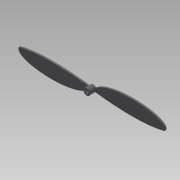
# Autodesk Inventor part: Helice 7x3
Saved by Autodesk Inventor 2016 (Build 200138000, 138)
## iProperties
Created: 2016-01-22
Part Number: Helice 7x3
Material: Plastique ABS
Document SubType Name: Modeling
Designer: sd
Density: 1.06 g/cm^3
Appearance: Lisse - Gris moyen
Mass: 5.43361 g
Surface Area: 59.4069 cm^2
Volume: 5.12605 cm^3
Author: sd
Autodesk Inventor part; units mm, degrees
ref_plane "YZ Plane" through (0, 0, 0) normal (1, 0, 0) x (0, 1, 0)
ref_plane "XZ Plane" through (0, 0, 0) normal (0, 1, 0) x (-1, 0, 0)
ref_plane "XY Plane" through (0, 0, 0) normal (0, 0, 1) x (1, 0, 0)
sketch "Esquisse4" plane through (0, 0, 0) normal (0, 1, 0) x (-1, 0, 0)
  circle A0 centre (0, 0) radius 2.25
  circle A1 centre (0, 0) radius 4
  dimension "d6" = 4.5
  dimension "d7" = 8
  constraints: 2 centre point, 2 coincident
  measures "d6" diameter of A0
  measures "d7" diameter of A1
extrude "Extrusion2" add sketch "Esquisse4" along normal blind 8
sketch "Esquisse5" plane through (0, 8, 0) normal (0, 1, 0) x (1, 0, 0)
  circle A0 centre (0, 0) radius 4 projected
  circle A1 centre (0, 0) radius 88.9
  spline S0 degree 3 poles (-88.9, 0) (-96.1137, 15.1507) (-22.3547, 20.9921) (-3.3072, 2.25) knots 0 0 0 0 1 1 1 1
  spline S1 degree 2 poles (-88.9, 0) (-58.1385, -7.7753) (-3.873, -1) knots 0 0 0 1 1 1
  point P0 (-86.0001, 7)
  point P1 (-47, 14)
  point P2 (-58, -4)
  dimension "d10" = 177.8
  constraints: 2 point on circle, 1 coincident, 1 horizontal alignment, 9 other
extrude "Extrusion3" add sketch "Esquisse5" against normal blind 2 contours A0 S1 A1 S0 | A1 S0 picked at (-43.854, 2.0054)
pattern_circular "Réseau circulaire1" count 2 over 360 about axis through (0, 0, 0) along (0, -1, 0) of "Extrusion3"
